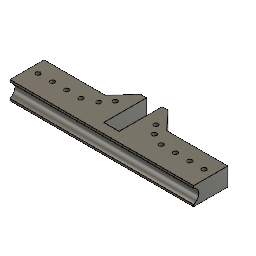
37part (Autodesk Fusion 360 design; units mm, degrees)
Autodesk Fusion 360 part; units mm, degrees
sketch "Sketch1" plane through (0, 0, 0) normal (0, 1, 0) x (1, 0, 0)
  line L0 (0, 0) -> (-75, 0)
  line L1 (-75, 0) -> (-75, 28)
  line L2 (-75, 28) -> (-25, 28)
  line L3 (-25, 28) -> (-11.25, 43)
  line L4 (-11.25, 43) -> (-6.25, 43)
  line L5 (-6.25, 43) -> (-6.25, 8)
  line L6 (-6.25, 8) -> (0, 8)
  line L7 (75, 28) -> (25, 28)
  line L8 (6.25, 43) -> (6.25, 8)
  line L9 (11.25, 43) -> (6.25, 43)
  line L10 (6.25, 8) -> (0, 8)
  line L11 (75, 0) -> (75, 28)
  line L12 (25, 28) -> (11.25, 43)
  line L13 (0, 0) -> (75, 0)
  line L14 (0, 55.2987) -> (0, -14.9715) construction
  dimension "d1" = 150
  dimension "d2" = 28
  dimension "d3" = 50
  dimension "d4" = 12.5
  dimension "d5" = 5
  dimension "d6" = 15
  dimension "d7" = 35
  constraint horizontal L0
  constraint perpendicular L0 L1
  constraint perpendicular L1 L2
  constraint perpendicular L1 L4
  constraint perpendicular L4 L5
  constraint perpendicular L5 L6
  constraint coincident L0.start L13.start
  constraint coincident L6.end L10.end
  constraint horizontal L7
  constraint horizontal L13
  constraint horizontal L10
  constraint equal L1 L11
  constraint equal L5 L8
  constraint equal L2 L7
  constraint equal L0 L13
  constraint equal L6 L10
  constraint equal L4 L9
  constraint vertical L14
  constraint coincident L0.start L14
  measures "d1" distance of L1 L11
  measures "d2" distance of L11.start L7.start
  measures "d3" distance of L1.end L2.end
  measures "d4" distance of L5 L8
  measures "d5" distance of L3.end L4.end
  measures "d6" distance of L7 L9
  measures "d7" distance of L8.end L8.start
extrude "Extrude1" add sketch "Sketch1" along normal mid plane 15
ref_plane "WorkPlane1" through (76, 0, -14) normal (1, 0, 0) x (0, 0, -1)
sketch "Sketch2" plane through (76, 7.5, -12.5) normal (1, 0, 0) x (0, 0, -1)
  circle A0 centre (-14.3163, -7.5683) radius 6
  dimension "d11" = 12
  measures "d11" diameter of A0
extrude "Extrude2" cut sketch "Sketch2" against normal through all
sketch "Sketch3" plane through (0, 0, 0) normal (0, 1, 0) x (1, 0, 0)
  circle A0 centre (-67.682, 16.9477) radius 1.75
  circle A1 centre (-56.0154, 16.9477) radius 1.75
  circle A2 centre (-44.3487, 16.9477) radius 1.75
  circle A3 centre (-32.682, 16.9477) radius 1.75
  circle A4 centre (-22.651, 21.2776) radius 1.75
  circle A5 centre (-16.5891, 28.4942) radius 1.75
  circle A6 centre (32.682, 16.9477) radius 1.75
  circle A7 centre (56.0154, 16.9477) radius 1.75
  circle A8 centre (44.3487, 16.9477) radius 1.75
  circle A9 centre (67.682, 16.9477) radius 1.75
  circle A10 centre (16.5891, 28.4942) radius 1.75
  circle A11 centre (22.651, 21.2776) radius 1.75
  line L0 (-70, -10) -> (65, -10) construction
  line L1 (0, 55.148) -> (0, -15.0653) construction
  dimension "d16" = 35
  dimension "d17" = 0
  dimension "d21" = 3.5
  constraint horizontal L0
  constraint vertical L1
  constraint coincident origin L1
  constraint symmetric A0.centre A9.centre L1
  constraint symmetric A1.centre A7.centre L1
  constraint symmetric A2.centre A8.centre L1
  constraint symmetric A3.centre A6.centre L1
  constraint symmetric A4.centre A11.centre L1
  constraint symmetric A5.centre A10.centre L1
  constraint equal A4 A5
  constraint equal A3 A5
  constraint equal A5 A6
  constraint equal A5 A9
  constraint equal A5 A7
  constraint equal A5 A8
  constraint equal A5 A11
  constraint equal A5 A10
  measures "d21" diameter of A5
revolve "Revolve1" cut sketch "Sketch3" angle 360 about axis through (-70, 0, 10) along (1, 0, 0)
